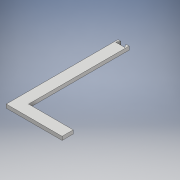
# Autodesk Inventor part: Liu_Inital_L
Saved by Autodesk Inventor 2017 (Build 210142000, 142)
## iProperties
Created: 2016-09-28
Part Number: Liu_Inital_L
Material: Generic
Document SubType Name: Modeling
Designer: jliu
Density: 1 g/cm^3
Appearance: Default
Author: jliu
Autodesk Inventor part; units mm, degrees
ref_plane "YZ Plane" through (0, 0, 0) normal (1, 0, 0) x (0, 1, 0)
ref_plane "XZ Plane" through (0, 0, 0) normal (0, 1, 0) x (-1, 0, 0)
ref_plane "XY Plane" through (0, 0, 0) normal (0, 0, 1) x (1, 0, 0)
sketch "Sketch1" plane through (0, 0, 0) normal (0, 0, 1) x (1, 0, 0)
  line L0 (5, -45) -> (5, 45)
  line L1 (-5, 45) -> (-5, -55)
  line L2 (-5, -55) -> (45, -55)
  line L3 (45, -55) -> (45, -45)
  line L4 (45, -45) -> (5, -45)
  line L5 (0, 45) -> (0, 42) construction
  line L6 (0, 42) -> (4, 42)
  line L7 (4, 42) -> (0, 42)
  line L8 (4, 42) -> (11.2559, 42) construction
  line L9 (4, 42) -> (2.2679, 45)
  line L10 (4, 42) -> (7.4641, 42) construction
  line L11 (0, 42) -> (-4, 42)
  line L12 (-4, 42) -> (-2.2679, 45)
  line L13 (-5, 45) -> (-2.2679, 45)
  line L14 (2.2679, 45) -> (5, 45)
  line L15 (2.2679, 45) -> (-2.2679, 45) construction
  point P0 (0, 0)
  dimension "d0" = 10
  dimension "d1" = 45
  dimension "d2" = 100
  dimension "d3" = 45
  dimension "d4" = 5
  dimension "d5" = 50
  dimension "d8" = 3
  dimension "d9" = 4
  dimension "d12" = 120
  dimension "d13" = 4
  dimension "d14" = 60
  dimension "d15" = 45
  dimension "d16" = 87
  dimension "d17" = 33.7441
  constraints: 32 end point, 4 perpendicular, 3 collinear, 3 horizontal, 2 vertical, 1 equal length, 1 parallel, 1 point on line
  measures "d0" distance of L0.end L1.start
  measures "d1" vertical distance of point (0, 0) L0.end
  measures "d2" distance of L1.end L1.start
  measures "d3" vertical distance of L0.start point (0, 0)
  measures "d4" distance from line of L1 point (0, 0)
  measures "d5" distance of L2.end L1.end
  measures "d8" distance of L5.start L5.end
  measures "d9" distance of L5.end L6.end
  measures "d12" angle of L10 L9
  measures "d13" distance of L5.end L11.end
  measures "d14" angle of L11 L12
  measures "d15" distance between parallel lines of L5 L3
  measures "d16" distance between parallel lines of L4 L6
  measures "d17" distance from line of L8.end L3
extrude "Extrusion1" add sketch "Sketch1" along normal mid plane 3.175
body "Solid1"
